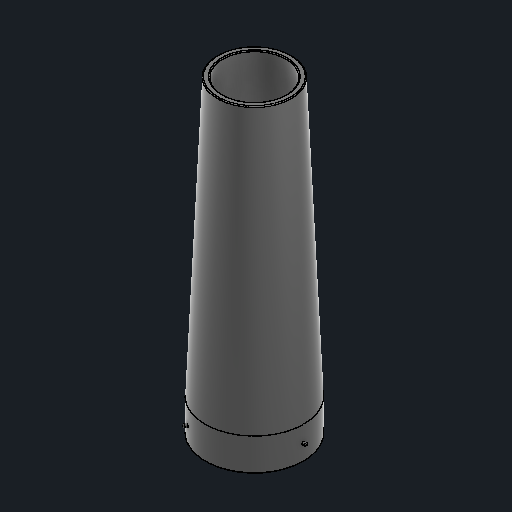
# Autodesk Inventor part: Tapered Vac Fitting
Saved by Autodesk Inventor 2026.2 (Build 302298000, 298)
## iProperties
Created: 2026-07-13
Part Number: Tapered Vac Fitting
Material: PVC, Unplasticized
Document SubType Name: Modeling
Designer: Joshua Eah
Density: 1.29 g/cm^3
Appearance: Smooth - Black
Author: Joshua Eah
Autodesk Inventor part; units mm, degrees
ref_plane "YZ Plane" through (0, 0, 0) normal (1, 0, 0) x (0, 1, 0)
ref_plane "XZ Plane" through (0, 0, 0) normal (0, 1, 0) x (-1, 0, 0)
ref_plane "XY Plane" through (0, 0, 0) normal (0, 0, 1) x (1, 0, 0)
sketch "Base Profile" plane through (0, 0, 0) normal (0, 1, 0) x (-1, 0, 0)
  circle A0 centre (0, 0) radius 22.5
  circle A1 centre (0, 0) radius 20
  dimension "d55" = 45
  dimension "d56" = 40
  constraints: 2 centre point, 2 coincident
  measures "d55" diameter of A0
  measures "d56" diameter of A1
extrude "Bayonet Mounting" add sketch "Base Profile" along normal blind 15
sketch "Sketch4" plane through (0, 0, 0) normal (0, 0, 1) x (1, 0, 0)
  line L0 (0, 0) -> (0, 15)
  line L1 (0, 15) -> (22.5, 15)
  line L2 (0, 0) -> (22.5, 0)
  line L3 (22.5, 15) -> (22.5, 0)
  line L4 (21, 8.25) -> (24, 8.25)
  line L5 (24, 8.25) -> (24, 6.75)
  line L6 (24, 6.75) -> (21, 6.75)
  line L7 (21, 6.75) -> (21, 8.25)
  line L8 (21, 8.25) -> (24, 6.75) construction
  line L9 (24, 8.25) -> (21, 6.75) construction
  line L10 (24, 7.5) -> (21, 7.5)
  line L11 (22.5, 15) -> (16.9551, 142)
  line L12 (16.9551, 142) -> (0, 142)
  line L13 (0, 142) -> (0, 15)
  line L14 (14.4527, 142) -> (19.9976, 15)
  point P0 (22.5, 7.5)
  dimension "d59" = 15
  dimension "d60" = 45
  dimension "d106" = 1.5
  dimension "d107" = 1.5
  dimension "d113" = 127
  dimension "d114" = 87.5
  dimension "d115" = 2.5
  constraints: 30 end point, 5 midpoint, 4 horizontal, 3 parallel, 2 point on line, 2 vertical, 1 coincident, 1 collinear, 1 perpendicular
  measures "d59" distance of L0.start L0.end
  measures "d60" diameter of L3 L0
  measures "d106" distance between parallel lines of L5 L3
  measures "d107" distance of L4.end L5.end
  measures "d113" distance from line of L1 L11.end
  measures "d114" angle of L1 L11
  measures "d115" distance between parallel lines of L11 L14
revolve "Lug" add sketch "Sketch4" angle 360 about axis through (24, 7.5, 0) along (-1, 0, 0) contours L10 L7 L4 L3 | L3 L4 L5 L10
fillet "Lug Fillet" radius 0.5 1 edges at (24, 6.75, 0)
pattern_circular "Lugs" count 3 over 360 about axis through (0, -10, 0) along (0, 1, 0) of "Lug", "Lug Fillet"
revolve "Revolution5" add sketch "Sketch4" angle 360 about axis through (0, 142, 0) along (0, -1, 0) contours L14 L12 L11 L1
fillet "Fillet7" radius 0.4 4 edges at (22.5, 0, 0) (20, 0, 0) (-14.4527, 142, 0) (-16.9551, 142, 0)
equation "\"d106\" = lugThickness"
equation "\"d107\" = lugThickness"
equation "\"lugThickness\" = 1.5"
body "Solid2"
